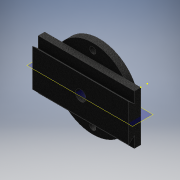
# Autodesk Inventor part: Top Part Tool bit
Saved by Autodesk Inventor 2016 (Build 200138000, 138)
## iProperties
Created: 2017-05-07
Part Number: Top Part Tool bit
Material: Steel, Cast
Document SubType Name: Modeling
Designer: Alex
Density: 7.85 g/cm^3
Appearance: Black Cast
Author: Alex
Autodesk Inventor part; units mm, degrees
ref_plane "YZ Plane" through (0, 0, 0) normal (1, 0, 0) x (0, 1, 0)
ref_plane "XZ Plane" through (0, 0, 0) normal (0, 1, 0) x (-1, 0, 0)
ref_plane "XY Plane" through (0, 0, 0) normal (0, 0, 1) x (1, 0, 0)
sketch "Sketch1" plane through (0, 0, 0) normal (1, 0, 0) x (0, 1, 0)
  line L0 (0, 0) -> (10.9, 0)
  line L1 (10.9, 0) -> (10.9, -85.6)
  line L2 (10.9, -85.6) -> (0, -85.6)
  line L3 (0, -85.6) -> (0, -66.6)
  line L4 (-10, -74.991) -> (-10, -10.609)
  line L5 (-10, -74.991) -> (0, -66.6)
  line L6 (0, 0) -> (0, -19)
  line L7 (0, -19) -> (-10, -10.609)
  line L8 (0, -66.6) -> (0, -19)
  line L9 (0, -42.8) -> (-10, -42.8) construction
  dimension "d1" = 85.6
  dimension "d7" = 19
  dimension "d30" = 50
  dimension "d31" = 19
  dimension "d32" = 50
  dimension "d33" = 10
  constraints: 20 end point, 3 perpendicular, 2 midpoint, 2 vertical, 1 horizontal, 1 parallel
  measures "d1" distance of L0.end L1.end
  measures "d7" distance of L0.start L6.end
  measures "d30" angle of L3 L5
  measures "d31" distance of L2.end L3.end
  measures "d32" angle of L6 L7
  measures "d33" distance between parallel lines of L8 L4
extrude "Extrusion1" add sketch "Sketch1" against normal blind 165.2
sketch "Sketch2" plane through (0, 10.9, 0) normal (0, 1, 0) x (1, 0, 0)
  point P0 (0, 0)
sketch "Sketch3" plane through (0, 10.9, 0) normal (0, 1, 0) x (1, 0, 0)
  line L0 (0, 0) -> (0, 85.6) projected
  line L1 (0, 42.8) -> (-14, 42.8)
  line L2 (-14, 42.8) -> (-82.3, 42.8)
  circle A0 centre (-82.3, 42.8) radius 68.3
  dimension "d10" = 14
  dimension "d11" = 68.3
  constraints: 4 end point, 2 horizontal, 1 coincident, 1 horizontal alignment, 1 midpoint, 2 other
  measures "d10" distance of L1.start L1.end
  measures "d11" distance of L1.end L2.end
extrude "Extrusion2" add sketch "Sketch3" along normal blind 11.5
sketch "Sketch4" plane through (-82.3, 22.4, -42.8) normal (0, 1, 0) x (1, 0, 0)
  circle A0 centre (0, 0) radius 9.15
  point P0 (82.3, -42.8)
  dimension "d14" = 18.3
  constraints: 1 centre point
  measures "d14" diameter of A0
extrude "Extrusion3" cut sketch "Sketch4" against normal blind 73.75
sketch "Sketch5" plane through (-82.3, 22.4, -42.8) normal (0, 1, 0) x (1, 0, 0)
  circle A0 centre (0, 0) radius 68.3 projected
  line L0 (0, 68.3) -> (0, 62.3)
  line L1 (0, -68.3) -> (0, -62.3)
  line L2 (0, 62.3) -> (0, 56.9)
  circle A1 centre (0, 56.9) radius 5.4
  line L3 (0, -62.3) -> (0, -56.9)
  line L4 (82.3, -32.191) -> (-82.9, -32.191) projected
  circle A2 centre (0, -56.9) radius 5.4
  point P0 (82.3, -42.8)
  dimension "d17" = 6
  dimension "d18" = 6
  dimension "d19" = 5.4
  dimension "d20" = 5.4
  constraints: 8 end point, 3 vertical, 2 coincident, 2 point on circle, 2 vertical alignment, 1 perpendicular, 4 other
  measures "d17" distance of L0.start L0.end
  measures "d18" distance of L1.start L1.end
  measures "d19" distance of L0.end L2.end
  measures "d20" distance of L1.end L3.end
extrude "Extrusion4" cut sketch "Sketch5" against normal blind 73.75 contours A1 | A2
sketch "Sketch6" plane through (-82.3, 22.4, -42.8) normal (0, 1, 0) x (1, 0, 0)
  point P0 (82.3, -42.8)
sketch "Sketch7" plane through (-82.3, 22.4, -42.8) normal (0, 1, 0) x (1, 0, 0)
  circle A0 centre (0, 0) radius 68.3 projected
  line L0 (68.3, 0) -> (61.4, 0)
  line L1 (61.4, 0) -> (50.6, 0)
  circle A1 centre (50.6, 0) radius 10.8
  point P0 (82.3, -42.8)
  dimension "d23" = 6.9
  dimension "d24" = 10.8
  constraints: 4 end point, 2 horizontal, 2 horizontal alignment, 1 coincident, 3 other
  measures "d23" distance of L0.start L0.end
  measures "d24" distance of L0.end L1.end
extrude "Extrusion5" cut sketch "Sketch7" against normal blind 6 contours A1
sketch "Sketch8" plane through (-31.7, 16.4, -42.8) normal (0, 1, 0) x (1, 0, 0)
  circle A0 centre (0, 0) radius 3.1
  point P0 (31.7, -42.8)
  dimension "d27" = 6.2
  constraints: 1 centre point
  measures "d27" diameter of A0
extrude "Extrusion6" cut sketch "Sketch8" against normal blind 22.8
ref_plane "Work Plane1" through (0, 0, -42.8) normal (0, 0, -1) x (-1, 0, 0)
body "Solid1"
